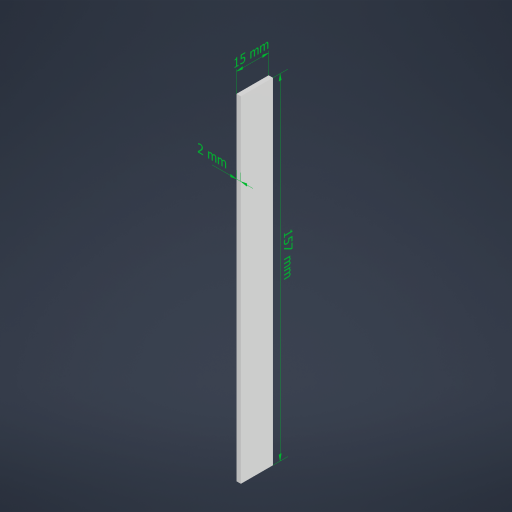
# Autodesk Inventor part: flat_bar
Saved by Autodesk Inventor 2023 (Build 270158000, 158)
## iProperties
Created: 2022-04-27
Part Number: flat_bar
Material: Aluminum 6061
Document SubType Name: Modeling
Designer: Norbert Ligas
Density: 2.7 g/cm^3
Appearance: Aluminum - Polished
Mass: 50.868 g
Surface Area: 84.04 cm^2
Volume: 18.84 cm^3
flat_bar_length: 157 mm
flat_bar_thickness: 2 mm
flat_bar_width: 15 mm
iron_angle_to_pipe_edge: 20 mm
pipe_length: 200,000 mm
pipe_outer_diameter: 12 mm
angle_iron_heigth: 15 mm
Author: Norbert Ligas
Autodesk Inventor part; units mm, degrees
ref_plane "YZ Plane" through (0, 0, 0) normal (1, 0, 0) x (0, 1, 0)
ref_plane "XZ Plane" through (0, 0, 0) normal (0, 1, 0) x (-1, 0, 0)
ref_plane "XY Plane" through (0, 0, 0) normal (0, 0, 1) x (1, 0, 0)
sketch "Sketch1" plane through (0, 0, 0) normal (0, 1, 0) x (-1, 0, 0)
  line L0 (1, 7.5) -> (-1, 7.5)
  line L1 (-1, 7.5) -> (-1, -7.5)
  line L2 (-1, -7.5) -> (1, -7.5)
  line L3 (1, -7.5) -> (1, 7.5)
  line L4 (0, -10.5) -> (0, 10.5) projected
  line L5 (-4.2, 0) -> (4.2, 0) projected
  point P0 (0, 0)
  dimension "d0" = 2
  dimension "d1" = 15
  constraints: 8 end point, 2 parallel, 1 horizontal, 1 perpendicular, 2 other
  measures "d0" distance of L1.end L2.end
  measures "d1" distance of L2.end L0.start
extrude "Extrusion1" add sketch "Sketch1" along normal blind 157
equation "\"d0\" = flat_bar_thickness"
equation "\"d1\" = flat_bar_width"
equation "\"d2\" = flat_bar_length"
equation "\"flat_bar_length\" = -2 * iron_angle_to_pipe_edge + pipe_length + pipe_outer_diameter - angle_iron_heigth"
equation "\"flat_bar_thickness\" = 2"
equation "\"flat_bar_width\" = 15"
equation "\"iron_angle_to_pipe_edge\" = 20"
equation "\"pipe_length\" = 200"
equation "\"pipe_outer_diameter\" = 12"
equation "\"angle_iron_heigth\" = 15"
body "Solid1"
